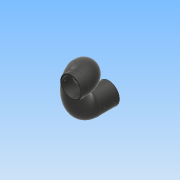
# Autodesk Inventor part: Top_Pipe 01
Saved by Autodesk Inventor 2018.1 (Build 221171000, 171)
## iProperties
Created: 2019-03-18
Part Number: Top_Pipe 01
Material: PVC-Piping
Document SubType Name: Modeling
Designer: James
Density: 1.4 g/cm^3
Appearance: Smooth - Black
Author: James
Autodesk Inventor part; units mm, degrees
ref_plane "XZ Plane" through (0, 0, 0) normal (0, 1, 0) x (-1, 0, 0)
ref_plane "XY Plane" through (0, 0, 0) normal (0, 0, 1) x (1, 0, 0)
sketch "Sketch1" plane through (0, 0, 0) normal (0, 1, 0) x (-1, 0, 0)
  circle A0 centre (0, 0) radius 23
  circle A1 centre (0, 0) radius 20
  dimension "d0" = 46
  dimension "d1" = 40
  constraints: 2 centre point, 2 coincident
  measures "d0" diameter of A0
  measures "d1" diameter of A1
sketch3d "3D Sketch1"
  spline S0 degree 4 poles (0, 0, 0) (0, -50, 0) (0, -50, 125) (74, -50, 125) (74, -100, 125) knots 1 1 1 1 1 2 2 2 2 2
  dimension "d31" = 50
  dimension "d32" = 125
  dimension "d33" = 74
  dimension "d34" = 50
sweep "Sweep1" add profiles "Sketch1" path "3D Sketch1"
sketch "Sketch2" plane through (0, 0, 0) normal (0, 1, 0) x (1, 0, 0)
  spline S0 degree 6 poles (-20, 0) (-20, 33.2309) (21.091, 38.0022) (54.9823, 0) (21.091, -38.0022) (-20, -33.2309) (-20, 0) knots 0 0 0 0 0 0 0 1 1 1 1 1 1 1 weights 1.669078 1.03673 1.038347 0.853534 1.038347 1.03673 1.669078 projected
  circle A0 centre (0, 0) radius 23 projected
  point P0 (-23, 0)
  constraints: 1 horizontal alignment, 1 other
extrude "Extrusion1" add sketch "Sketch2" along normal blind 40
sketch "Sketch3" plane through (74, -100, 125) normal (0, -1, 0) x (1, 0, 0)
  spline S0 degree 6 poles (-14.7842, 13.4695) (-37.1644, -11.095) (-10.003, -42.2959) (40.6434, -37.0293) (41.1842, 13.8873) (7.596, 38.0341) (-14.7842, 13.4695) knots 0 0 0 0 0 0 0 1 1 1 1 1 1 1 weights 1.669078 1.03673 1.038347 0.853534 1.038347 1.03673 1.669078 projected
  circle A0 centre (0, 0) radius 23 projected
  point P0 (-74, -125)
  point P1 (-16.5141, 16.0089)
  constraints: 2 other
extrude "Extrusion2" add sketch "Sketch3" along normal blind 15 contours S0 picked at (-15.0218, 15.8833)
ref_plane "Work Plane1" through (74, 0, 0) normal (1, 0, 0) x (0, 1, 0)
sketch "Sketch4" plane through (74, 0, 0) normal (1, 0, 0) x (0, 1, 0)
  line L0 (-115, 145) -> (-115, 105) projected
  line L1 (-100, 138.9208) -> (-100, 145) projected
  point P0 (0, 0)
  point P1 (-107.5, 125)
  point P2 (-115, 138.9208)
  dimension "d12" = 7.5
  dimension "d13" = -20
  dimension "d14" = 20
  measures "d12" distance from line of L0 point (-107.5, 125)
  measures "d13" vertical distance of point (-107.5, 125) L0.end
  measures "d14" vertical distance of L0.start point (-107.5, 125)
hole "Hole1" at (74, -107.5, 125) direction (-1, 0, 0) diameter 4.5 end through all
sketch "Sketch5" plane through (0, 0, 0) normal (1, 0, 0) x (0, 1, 0)
  line L0 (40, -20) -> (40, 20) projected
  point P0 (0, 0)
  point P1 (30, 0)
  point P2 (10, 0)
  point P3 (40, 0)
  point P4 (40, 0)
  dimension "d22" = 10
  dimension "d23" = 20
  constraints: 2 horizontal alignment, 1 midpoint
  measures "d22" distance from line of point (30, 0) L0
  measures "d23" distance of point (10, 0) point (30, 0)
hole "Hole2" at (0, 30, 0) at (0, 10, 0) direction (1, 0, 0) diameter 4.5 end through all
body "Solid1"
